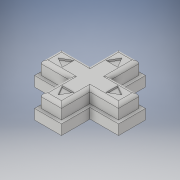
# Autodesk Inventor part: Kreuz
Saved by Autodesk Inventor 2019 (Build 230136000, 136)
## iProperties
Created: 2020-09-25
Part Number: Kreuz
Material: Generisch
Document SubType Name: Modeling
Designer: David
Density: 1 g/cm^3
Appearance: Vorgabe
Author: David
Autodesk Inventor part; units mm, degrees
ref_plane "YZ Plane" through (0, 0, 0) normal (1, 0, 0) x (0, 1, 0)
ref_plane "XZ Plane" through (0, 0, 0) normal (0, 1, 0) x (-1, 0, 0)
ref_plane "XY Plane" through (0, 0, 0) normal (0, 0, 1) x (1, 0, 0)
sketch "Skizze1" plane through (0, 0, 0) normal (0, 1, 0) x (-1, 0, 0)
  line L0 (0, 0) -> (0, -8.5)
  line L1 (0, -8.5) -> (8.5, -8.5)
  line L2 (8.5, -8.5) -> (8.5, -14.5)
  line L3 (8.5, -14.5) -> (0, -14.5)
  line L4 (0, -14.5) -> (0, -23)
  line L5 (0, -23) -> (-6, -23)
  line L6 (-6, -23) -> (-6, -14.5)
  line L7 (-6, -14.5) -> (-14.5, -14.5)
  line L8 (-14.5, -14.5) -> (-14.5, -8.5)
  line L9 (-14.5, -8.5) -> (-6, -8.5)
  line L10 (-6, 0) -> (0, 0)
  line L11 (-6, -8.5) -> (-6, 0)
  dimension "d0" = 23
  dimension "d1" = 23
  dimension "d2" = 6
  dimension "d3" = 6
  dimension "d4" = 8.5
  dimension "d5" = 8.5
  dimension "d6" = 8.5
  constraints: 24 end point, 8 point on line, 6 perpendicular, 2 vertical, 1 parallel
  measures "d0" distance between parallel lines of L5 L10
  measures "d1" distance between parallel lines of L8 L2
  measures "d2" distance of L1.end L2.end
  measures "d3" distance of L4.end L5.end
  measures "d4" distance of L0.end L1.end
  measures "d5" distance of L8.end L9.end
  measures "d6" distance of L3.end L4.end
extrude "Extrusion1" add sketch "Skizze1" along normal blind 4
sketch "Skizze2" plane through (0, 4, 0) normal (0, 1, 0) x (1, 0, 0)
  line L0 (3, 1.9793) -> (1.25, 5.0104)
  line L1 (1.25, 5.0104) -> (4.75, 5.0104)
  line L2 (4.75, 5.0104) -> (3, 1.9793)
  line L3 (6, 23) -> (0, 23) projected
  line L4 (0, 0) -> (6, 0) projected
  line L5 (3, 21.0207) -> (4.75, 17.9896)
  line L6 (4.75, 17.9896) -> (1.25, 17.9896)
  line L7 (1.25, 17.9896) -> (3, 21.0207)
  line L8 (-6.5207, 11.5) -> (-3.4896, 13.25)
  line L9 (-3.4896, 13.25) -> (-3.4896, 9.75)
  line L10 (-3.4896, 9.75) -> (-6.5207, 11.5)
  line L11 (12.5207, 11.5) -> (9.4896, 9.75)
  line L12 (9.4896, 9.75) -> (9.4896, 13.25)
  line L13 (9.4896, 13.25) -> (12.5207, 11.5)
  line L14 (-8.5, 14.5) -> (-8.5, 8.5) projected
  line L15 (14.5, 8.5) -> (14.5, 14.5) projected
  point P0 (3, 4)
  point P1 (3, 19)
  point P2 (-4.5, 11.5)
  point P3 (10.5, 11.5)
  dimension "d9" = 4
  dimension "d10" = 3
  dimension "d11" = 4
  dimension "d12" = 4
  dimension "d13" = 4
  dimension "d14" = 3
  dimension "d15" = 3
  dimension "d16" = 3
  dimension "d17" = 3.5
  dimension "d18" = 3.5
  dimension "d19" = 3.5
  dimension "d20" = 3.5
  constraints: 24 end point, 4 parallel, 28 other
  measures "d9" distance from line of L4 point (3, 4)
  measures "d10" horizontal distance of L4.start point (3, 4)
  measures "d11" horizontal distance of L15.start point (10.5, 11.5)
  measures "d12" distance from line of L3 point (3, 19)
  measures "d13" distance from line of L14 point (-4.5, 11.5)
  measures "d14" vertical distance of L14.end point (-4.5, 11.5)
  measures "d15" horizontal distance of L3.end point (3, 19)
  measures "d16" vertical distance of L15.start point (10.5, 11.5)
  measures "d17" distance of L0.end L1.end
  measures "d18" distance of L5.end L6.end
  measures "d19" distance of L8.end L9.end
  measures "d20" distance of L11.end L12.end
extrude "Extrusion2" cut sketch "Skizze2" against normal blind 0.5
fillet "Rundung1" radius 1 12 edges at (6, 4, -4.25) (3, 4, 0) (0, 4, -4.25) (10.25, 4, -8.5) (10.25, 4, -14.5) (14.5, 4, -11.5) (6, 4, -18.75) (3, 4, -23) (0, 4, -18.75) (-4.25, 4, -14.5) (-8.5, 4, -11.5) (-4.25, 4, -8.5)
sketch "Skizze3" plane through (0, 0, 0) normal (0, -1, 0) x (1, 0, 0)
  line L0 (15.5, -15.5) -> (7, -15.5)
  line L1 (7, -15.5) -> (7, -24)
  line L2 (7, -24) -> (-1, -24)
  line L3 (-1, -24) -> (-1, -15.5)
  line L4 (-1, -15.5) -> (-9.5, -15.5)
  line L5 (-9.5, -15.5) -> (-9.5, -7.5)
  line L6 (-9.5, -7.5) -> (-1, -7.5)
  line L7 (-1, -7.5) -> (-1, 1)
  line L8 (-1, 1) -> (7, 1)
  line L9 (7, 1) -> (7, -7.5)
  line L10 (14.5, -8.5) -> (6, -8.5) projected
  line L11 (7, -7.5) -> (15.5, -7.5)
  line L12 (15.5, -7.5) -> (15.5, -15.5)
  point P0 (0, 0)
  point P1 (14.5, -14.5)
  point P2 (6, -23)
  point P3 (-8.5, -8.5)
  point P4 (0, -8.5)
  point P5 (6, 0)
  dimension "d25" = 8.5
  dimension "d26" = 25
  dimension "d27" = 25
  dimension "d28" = 8
  dimension "d29" = 8
  dimension "d30" = 8
  dimension "d31" = 8
  dimension "d32" = 8.5
  dimension "d33" = 8.5
  dimension "d34" = 8.5
  dimension "d35" = 8.5
  dimension "d36" = 8.5
  constraints: 24 end point, 5 perpendicular, 1 parallel, 1 vertical
  measures "d25" distance of L8.end L9.end
  measures "d26" distance between parallel lines of L5 L12
  measures "d27" distance between parallel lines of L8 L2
  measures "d28" distance of L4.end L5.end
  measures "d29" distance of L1.end L2.end
  measures "d30" distance of L11.end L0.start
  measures "d31" distance of L7.end L8.end
  measures "d32" distance of L9.end L11.end
  measures "d33" distance of L5.end L6.end
  measures "d34" distance of L3.end L4.end
  measures "d35" distance of L0.start L0.end
  measures "d36" distance of L6.end L7.end
extrude "Extrusion3" add sketch "Skizze3" along normal blind 3
